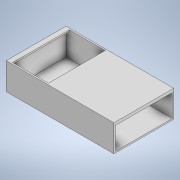
# Autodesk Inventor part: ShootingMech_Housing3
Saved by Autodesk Inventor 2020 (Build 240168000, 168)
## iProperties
Created: 2021-12-09
Part Number: ShootingMech_Housing3
Material: Generic
Document SubType Name: Modeling
Designer: danie
Density: 1 g/cm^3
Appearance: Default
Author: danie
Autodesk Inventor part; units mm, degrees
ref_plane "YZ Plane" through (0, 0, 0) normal (1, 0, 0) x (0, 1, 0)
ref_plane "XZ Plane" through (0, 0, 0) normal (0, 1, 0) x (-1, 0, 0)
ref_plane "XY Plane" through (0, 0, 0) normal (0, 0, 1) x (1, 0, 0)
sketch "Sketch1" plane through (0, 0, 0) normal (0, 1, 0) x (-1, 0, 0)
  line L0 (0, 0) -> (-228.6, 0)
  line L1 (-228.6, 0) -> (-228.6, 127)
  line L2 (-228.6, 127) -> (0, 127)
  line L3 (0, 127) -> (0, 0)
  dimension "d0" = 228.6
  dimension "d1" = 127
  constraints: 8 end point, 2 parallel, 1 horizontal, 1 perpendicular
  measures "d0" distance of L1.end L2.end
  measures "d1" distance of L0.end L1.end
extrude "Extrusion1" add sketch "Sketch1" along normal blind 3.175
sketch "Sketch2" plane through (0, 3.175, 0) normal (0, 1, 0) x (1, 0, 0)
  line L0 (228.6, 0) -> (0, 0) projected
  line L1 (0, -127) -> (228.6, -127) projected
  line L2 (0, 0) -> (228.6, 0)
  line L3 (228.6, -127) -> (0, -127)
  line L4 (0, -127) -> (0, 0)
  line L5 (0, 0) -> (0, -127) projected
  line L6 (0, 0) -> (228.6, 0)
  line L7 (228.6, 0) -> (228.6, -127)
  line L8 (228.6, -127) -> (0, -127)
  line L9 (0, -127) -> (0, 0)
  line L10 (228.6, -3.175) -> (3.175, -3.175)
  line L11 (3.175, -3.175) -> (3.175, -123.825)
  line L12 (3.175, -123.825) -> (228.6, -123.825)
  dimension "d4" = 3.175
  constraints: 20 end point, 3 parallel, 2 horizontal, 1 perpendicular, 2 other
  measures "d4" distance between parallel lines of L0 L10
extrude "Extrusion2" add sketch "Sketch2" along normal blind 50.8 contours L7 L10 L11 L12 L1 L4 L0
sketch "Sketch3" plane through (228.6, 0, 127) normal (1, 0, 0) x (0, 0, -1)
  line L0 (127, 53.975) -> (0, 53.975) projected
  line L1 (0, 53.975) -> (127, 53.975)
  line L2 (127, 53.975) -> (127, 0)
  line L3 (127, 0) -> (0, 0)
  line L4 (0, 0) -> (0, 53.975)
  line L5 (3.175, 50.8) -> (123.825, 50.8)
  line L6 (123.825, 50.8) -> (123.825, 3.175)
  line L7 (123.825, 3.175) -> (3.175, 3.175)
  line L8 (3.175, 3.175) -> (3.175, 50.8)
  dimension "d7" = 3.175
  constraints: 16 end point, 4 parallel, 2 perpendicular, 1 horizontal, 3 other
  measures "d7" distance between parallel lines of L4 L8
extrude "Extrusion3" add sketch "Sketch3" against normal blind 3.175
sketch "Sketch4" plane through (0, 53.975, 0) normal (0, 1, 0) x (1, 0, 0)
  line L0 (228.6, 0) -> (0, 0) projected
  line L1 (0, -127) -> (228.6, -127) projected
  line L2 (0, 0) -> (228.6, 0)
  line L3 (228.6, 0) -> (228.6, -127)
  line L4 (228.6, -127) -> (0, -127)
  line L5 (0, -127) -> (0, 0)
  line L6 (3.175, -123.825) -> (228.6, -123.825) construction
  line L7 (3.175, -123.825) -> (79.375, -123.825) construction
  line L8 (228.6, -127) -> (228.6, 0) projected
  line L9 (79.375, -123.825) -> (228.6, -123.825)
  line L10 (228.6, -123.825) -> (228.6, 0)
  line L11 (228.6, 0) -> (79.375, 0)
  line L12 (3.175, -123.825) -> (3.175, -3.175) projected
  line L13 (3.175, -3.175) -> (79.375, -3.175)
  line L14 (79.375, -123.825) -> (3.175, -123.825)
  line L15 (3.175, -123.825) -> (3.175, -3.175)
  line L16 (79.375, -3.175) -> (155.575, -3.175)
  line L17 (155.575, -123.825) -> (79.375, -123.825)
  line L18 (3.175, -123.825) -> (117.475, -123.825) construction
  line L19 (225.425, -123.825) -> (3.175, -123.825) construction
  line L20 (117.475, -123.825) -> (41.275, -123.825)
  line L21 (41.275, -3.175) -> (117.475, -3.175)
  line L22 (3.175, -3.175) -> (225.425, -3.175) projected
  line L23 (10.1575, -3.175) -> (86.3575, -3.175)
  line L24 (86.3575, -3.175) -> (86.3575, -123.825)
  line L25 (86.3575, -123.825) -> (10.1575, -123.825)
  line L26 (10.1575, -123.825) -> (10.1575, -3.175)
  point P0 (10.1575, -123.825)
  dimension "d10" = 76.2
  dimension "d13" = 76.2
  dimension "d15" = 114.3
  dimension "d16" = 76.2
  dimension "d17" = 76.2
  constraints: 40 end point, 8 parallel, 6 horizontal, 5 point on line, 3 perpendicular, 1 midpoint
  measures "d10" distance of L6.start L7.end
  measures "d13" distance of L17.start L17.end
  measures "d15" distance of L14.end L18.end
  measures "d16" distance of L21.start L21.end
  measures "d17" distance of L24.end L25.end
extrude "Extrusion4" add sketch "Sketch4" along normal blind 3.175 contours L3 L1 L5 L0 | L14 L12 L13 L26
body "Solid1"
